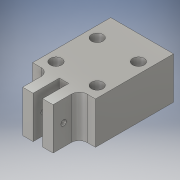
# Autodesk Inventor part: Mass 1 V2
Saved by Autodesk Inventor 2016 (Build 200138000, 138)
## iProperties
Created: 2015-07-10
Part Number: Mass 1 V2
Material: Aluminum 6061
Document SubType Name: Modeling
Designer: Dennis
Density: 2.7 g/cm^3
Appearance: Aluminum - Polished
Author: Dennis
Autodesk Inventor part; units mm, degrees
ref_plane "YZ Plane" through (0, 0, 0) normal (1, 0, 0) x (0, 1, 0)
ref_plane "XZ Plane" through (0, 0, 0) normal (0, 1, 0) x (-1, 0, 0)
ref_plane "XY Plane" through (0, 0, 0) normal (0, 0, 1) x (1, 0, 0)
sketch "Sketch1" plane through (0, 0, 0) normal (0, 1, 0) x (-1, 0, 0)
  line L0 (-38.1, 47.35) -> (38.1, 47.35)
  line L1 (38.1, 47.35) -> (38.1, -47.35)
  line L2 (38.1, -47.35) -> (-38.1, -47.35)
  line L3 (-38.1, -47.35) -> (-38.1, 47.35)
  line L4 (-38.1, 47.35) -> (38.1, -47.35) construction
  line L5 (38.1, 47.35) -> (-38.1, -47.35) construction
  point P0 (0, 0)
  dimension "d0" = 76.2
  dimension "d1" = 94.7
  constraints: 12 end point, 2 midpoint, 2 parallel, 1 horizontal, 1 perpendicular
  measures "d0" distance of L1.end L2.end
  measures "d1" distance of L0.end L1.end
extrude "Block" add sketch "Sketch1" along normal blind 50.8
sketch "Sketch2" plane through (0, 0, 0) normal (0, 1, 0) x (-1, 0, 0)
  line L0 (38.1, 47.35) -> (-38.1, 47.35) projected
  line L1 (18.415, 47.35) -> (5.715, 47.35)
  line L2 (5.715, 47.35) -> (5.715, 79.1)
  line L3 (5.715, 79.1) -> (18.415, 79.1)
  line L4 (18.415, 79.1) -> (18.415, 47.35)
  line L5 (-5.715, 47.35) -> (-18.415, 47.35)
  line L6 (-18.415, 47.35) -> (-18.415, 79.1)
  line L7 (-18.415, 79.1) -> (-5.715, 79.1)
  line L8 (-5.715, 79.1) -> (-5.715, 47.35)
  line L9 (38.1, 47.35) -> (18.415, 47.35) construction
  line L10 (-18.415, 47.35) -> (-38.1, 47.35) construction
  point P0 (0, 0)
  dimension "d4" = 12.7
  dimension "d5" = 11.43
  dimension "d17" = 31.75
  constraints: 20 end point, 4 parallel, 3 equal length, 2 collinear, 2 horizontal, 2 perpendicular, 2 point on line
  measures "d4" distance of L2.end L3.end
  measures "d5" distance between parallel lines of L8 L2
  measures "d17" distance of L3.end L1.start
extrude "Tabs" add sketch "Sketch2" along normal up to surface (50.8 mm away)
hole "Arm Mounting Hole" at (18.415, 25.4, 66.4) direction (-1, 0, 0) diameter 6.5278 end up to face face through (-18.415, 33.8667, 57.9333) facing (-1, 0, 0)
hole "Mounting Hole" at (-24.9936, 50.8, 32.1608) direction (0, -1, 0) diameter 8 end up to face face through (-1.905, 0, -15.7833) facing (0, -1, 0) counterbore diameter 14 counterbore depth 30.48
pattern_linear "Mounting Holes" count 2 spacing 50 along (0, 0, -1) count 2 spacing 50 along (1, 0, 0) of "Mounting Hole"
hole "Spring Hole" at (3.1, 25.4, -47.35) direction (0, 0, 1) diameter 4.1402 depth 12.7 tip angle 118
fillet "Fillet1" radius 9.525 2 edges at (18.415, 25.4, 47.35) (-18.415, 25.4, 47.35)
body "Solid1"
